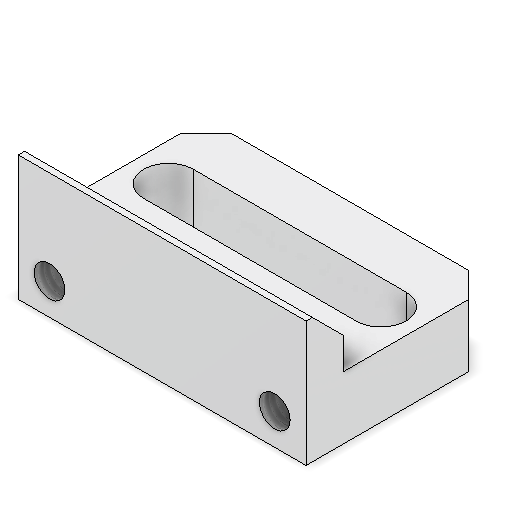
# Autodesk Inventor part: SUPORTE ADAPTADOR USB TIPO C REV03 - PARTE 02
Saved by Autodesk Inventor 2025.1 (Build 291241020, 241B)
## iProperties
Created: 2025-03-19
Part Number: SUPORTE ADAPTADOR USB TIPO C REV03 - PARTE 02
Material: Alumínio 6061
Document SubType Name: Modeling
Designer: Thiago Fortes
Density: 2.7 g/cm^3
Appearance: Alumínio - Plano
Description: SUPORTE ADAPTADOR USB TIPO C REV03 - PARTE 02
Author: Thiago Fortes
Autodesk Inventor part; units mm, degrees
ref_plane "YZ Plane" through (0, 0, 0) normal (1, 0, 0) x (0, 1, 0)
ref_plane "XZ Plane" through (0, 0, 0) normal (0, 1, 0) x (-1, 0, 0)
ref_plane "XY Plane" through (0, 0, 0) normal (0, 0, 1) x (1, 0, 0)
sketch "Esboço1" plane through (0, 0, 0) normal (0, 0, 1) x (1, 0, 0)
  line L0 (-11.5, 5) -> (11.5, 5)
  line L1 (11.5, 5) -> (11.5, -5)
  line L2 (11.5, -5) -> (-11.5, -5)
  line L3 (-11.5, -5) -> (-11.5, 5)
  line L4 (-11.5, 5) -> (11.5, -5) construction
  line L5 (11.5, 5) -> (-11.5, -5) construction
  point P0 (0, 0)
  dimension "d0" = 10
  dimension "d1" = 23
  constraints: 12 end point, 2 midpoint, 2 parallel, 1 horizontal, 1 perpendicular
  measures "d0" distance of L0.end L1.end
  measures "d1" distance of L0.start L0.end
extrude "Extrusão1" add sketch "Esboço1" along normal blind 15
chamfer "Chanfro1" distance 2 angle 45 2 edges at (-11.5, 0, 0) (11.5, 0, 0)
sketch "Esboço4" plane through (-11.5, -5, 15) normal (0, -1, 0) x (1, 0, 0)
  line L0 (11.5, -15) -> (11.5, -9)
  line L1 (3, -9) -> (20, -9) construction
  line L2 (3, -11) -> (20, -11)
  line L3 (20, -7) -> (3, -7)
  arc A0 (3, -7) -> (3, -11) centre (3, -9) ccw
  arc A1 (20, -11) -> (20, -7) centre (20, -9) ccw
  line L4 (23, -13) -> (23, 0) projected
  dimension "d18" = 6
  dimension "d19" = 4
  dimension "d20" = 3
  constraints: 10 end point, 4 point on circle, 4 tangent, 2 centre point, 1 horizontal, 1 midpoint, 1 parallel, 1 vertical
  measures "d18" distance of L0.start L0.end
  measures "d19" distance between parallel lines of L3 L2
  measures "d20" distance from line of L4 L1.end
extrude "Extrusão3" cut sketch "Esboço4" against normal through all
sketch "Esboço2" plane through (0, 0, 15) normal (0, 0, 1) x (1, 0, 0)
  line L0 (11.5, 5) -> (-11.5, 5) projected
  line L1 (-11.5, -5) -> (11.5, -5) projected
  line L2 (-9, -2.5) -> (9, -2.5)
  line L3 (0, 0) -> (0, -2.5)
  line L4 (-11.5, 5) -> (-11.5, -5) projected
  dimension "d32" = 2.5
  dimension "d36" = 2.5
  constraints: 4 end point, 1 coincident, 1 horizontal, 1 midpoint, 1 vertical
  measures "d32" distance between parallel lines of L1 L2
  measures "d36" distance from line of L4 L2.start
hole "Furo1" at (-9, -2.5, 15) at (9, -2.5, 15) direction (0, 0, -1) diameter 2.459 depth 7.5 tip angle 118 thread size "M3x0.5" class "6H" standard "ISO Metric profile"
sketch "Esboço5" plane through (0, 0, 0) normal (1, 0, 0) x (0, 1, 0)
  line L0 (5, 0) -> (-5, 0) projected
  line L1 (5, 0) -> (0, 0)
  line L2 (0, 0) -> (0, 12)
  line L3 (0, 12) -> (5, 12)
  line L4 (5, 12) -> (5, 0)
  line L5 (-5, 0) -> (-5, 2) projected
  line L6 (5, 15) -> (-5, 15) projected
  point P0 (0, 0)
  point P1 (2.5, 0)
  dimension "d27" = 5
  dimension "d29" = 3
  constraints: 8 end point, 2 parallel, 1 horizontal, 1 midpoint, 1 perpendicular
  measures "d27" distance between parallel lines of L5 L2
  measures "d29" distance between parallel lines of L6 L3
extrude "Extrusão4" cut sketch "Esboço5" along normal through all both and the other way through all
chamfer "Chanfro2" distance 2.5 angle 45 1 edges at (0, 5, 12)
